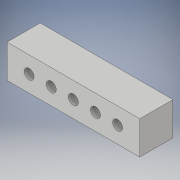
# Autodesk Inventor part: Splitter
Saved by Autodesk Inventor 2018 (Build 220112000, 112)
## iProperties
Created: 2020-03-28
Part Number: Splitter
Material: Generic
Document SubType Name: Modeling
Designer: emile
Density: 1 g/cm^3
Appearance: Default
Author: emile
Autodesk Inventor part; units mm, degrees
ref_plane "YZ Plane" through (0, 0, 0) normal (1, 0, 0) x (0, 1, 0)
ref_plane "XZ Plane" through (0, 0, 0) normal (0, 1, 0) x (-1, 0, 0)
ref_plane "XY Plane" through (0, 0, 0) normal (0, 0, 1) x (1, 0, 0)
sketch "Sketch1" plane through (0, 0, 0) normal (0, 0, 1) x (1, 0, 0)
  line L0 (76.2, -19.05) -> (-76.2, -19.05)
  line L1 (-76.2, -19.05) -> (-76.2, 19.05)
  line L2 (-76.2, 19.05) -> (76.2, 19.05)
  line L3 (76.2, 19.05) -> (76.2, -19.05)
  line L4 (76.2, -19.05) -> (-76.2, 19.05) construction
  line L5 (-76.2, -19.05) -> (76.2, 19.05) construction
  circle A0 centre (0, 0) radius 5.715
  dimension "d0" = 11.43
  dimension "d1" = 38.1
  dimension "d2" = 152.4
  constraints: 12 end point, 2 midpoint, 2 parallel, 1 centre point, 1 coincident, 1 horizontal, 1 perpendicular
  measures "d0" diameter of A0
  measures "d1" distance of L2.end L0.start
  measures "d2" distance of L1.end L2.end
extrude "Extrusion1" add sketch "Sketch1" along normal mid plane 38.1 contours L0 L1 L2 L3 | A0
extrude "Extrusion2" cut sketch "Sketch1" along normal through all contours A0
pattern_linear "Rectangular Pattern1" count 5 spacing 25.4 along (1, 0, 0) of "Extrusion2" first direction both ways yes
sketch "Sketch2" plane through (-76.2, -19.05, 19.05) normal (-1, 0, 0) x (0, 0, 1)
  circle A0 centre (-19.05, 19.05) radius 5.715
  dimension "d10" = 11.43
  constraints: 1 centre point, 1 coincident
  measures "d10" diameter of A0
extrude "Extrusion3" cut sketch "Sketch2" against normal blind 139.7
body "Solid1"
